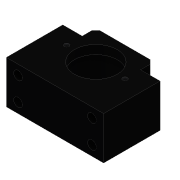
# Autodesk Inventor part: Lagerbock_Loslager
Saved by Autodesk Inventor 2016 (Build 200138000, 138)
## iProperties
Created: 2015-07-24
Part Number: Lagerbock_Loslager
Material: Aluminum 6061
Document SubType Name: Modeling
Density: 2.71 g/cm^3
Appearance: Smooth - Black
Autodesk Inventor part; units mm, degrees
ref_plane "YZ Plane" through (0, 0, 0) normal (1, 0, 0) x (0, 1, 0)
ref_plane "XZ Plane" through (0, 0, 0) normal (0, 1, 0) x (-1, 0, 0)
ref_plane "XY Plane" through (0, 0, 0) normal (0, 0, 1) x (1, 0, 0)
sketch "Sketch1" plane through (0, 0, 0) normal (0, 0, 1) x (1, 0, 0)
  line L0 (-25, 0) -> (25, 0)
  line L1 (25, 0) -> (25, 29)
  line L2 (25, 29) -> (15, 29)
  line L3 (15, 29) -> (15, 36)
  line L4 (15, 36) -> (-15, 36)
  line L5 (-15, 36) -> (-15, 29)
  line L6 (-15, 29) -> (-25, 29)
  line L7 (-25, 29) -> (-25, 0)
  point P0 (0, 0)
  point P1 (0, 0)
  dimension "d0" = 50
  dimension "d1" = 36
  dimension "d2" = 7
  dimension "d3" = 30
  constraints: 16 end point, 6 perpendicular, 2 point on line, 1 coincident, 1 collinear, 1 horizontal, 1 midpoint
  measures "d0" distance between parallel lines of L1 L7
  measures "d1" distance between parallel lines of L0 L4
  measures "d2" distance between parallel lines of L6 L4
  measures "d3" distance of L3.end L4.end
extrude "Extrusion1" add sketch "Sketch1" along normal mid plane 22
sketch "Sketch2" plane through (0, 0, 11) normal (0, 0, 1) x (1, 0, 0)
  line L0 (-25, 0) -> (25, 0) projected
  point P0 (0, 0)
  point P1 (0, 21)
  point P2 (0, 0)
  dimension "d6" = 21
  constraints: 1 midpoint, 1 vertical alignment
  measures "d6" distance from line of L0 point (0, 21)
hole "Hole1" at (0, 21, 11) direction (0, 0, -1) diameter 22 end through all
chamfer "Chamfer2" distance 2 angle 45 2 edges at (-15, 36, 0) (15, 36, 0)
sketch "Sketch3" plane through (-25, 29, 11) normal (0, 1, 0) x (1, 0, 0)
  line L0 (0, 22) -> (0, 0) projected
  line L1 (50, 22) -> (50, 0) projected
  line L2 (50, 22) -> (0, 22) projected
  line L3 (0, 0) -> (50, 0) projected
  point P0 (25, 11)
  point P1 (6, 17)
  point P2 (44, 17)
  point P3 (6, 5)
  point P4 (44, 5)
  dimension "d20" = 38
  dimension "d21" = 6
  dimension "d22" = 6
  dimension "d49" = 12
  dimension "d50" = 5
  dimension "d51" = 5
  constraints: 2 horizontal alignment, 2 vertical alignment
  measures "d20" distance of point (44, 17) point (6, 17)
  measures "d21" distance from line of L0 point (6, 17)
  measures "d22" distance from line of L1 point (44, 17)
  measures "d49" distance of point (6, 5) point (6, 17)
  measures "d50" distance from line of L2 point (6, 17)
  measures "d51" distance from line of L3 point (6, 5)
hole "Hole2" at (-19, 29, -6) at (19, 29, -6) at (-19, 29, 6) at (19, 29, 6) direction (0, -1, 0) diameter 4.5 end through all counterbore diameter 8 counterbore depth 5
sketch "Sketch5" plane through (0, 0, 11) normal (0, 0, 1) x (1, 0, 0)
  circle A0 centre (0, 21) radius 11 projected
  point P0 (0, 0)
  point P1 (-15, 21)
  point P2 (15, 21)
  dimension "d40" = 30
  dimension "d52" = 15
  constraints: 1 centre point, 1 horizontal alignment
  measures "d40" distance of point (15, 21) point (-15, 21)
  measures "d52" distance of point (15, 21) A0.centre
hole "Hole4" at (-15, 21, 11) at (15, 21, 11) direction (0, 0, -1) diameter 2.459 depth 10 tip angle 118 thread size "M3x0.5" designation "M3" class "6H" standard "ISO Metric profile"
hole "Hole5" at (0, 21, -11) direction (0, 0, 1) diameter 26 depth 17.5
sketch "Sketch6" plane through (0, 0, -11) normal (0, 0, -1) x (-1, 0, 0)
  circle A0 centre (0, 21) radius 15.5563 construction
  circle A1 centre (0, 21) radius 13 construction
  point P0 (0, 0)
  point P1 (-11, 32)
  point P2 (-11, 10)
  point P3 (11, 10)
  point P4 (11, 32)
  dimension "d62" = 22
  dimension "d63" = 22
  constraints: 4 point on circle, 2 horizontal alignment, 2 vertical alignment, 1 centre point, 1 concentric
  measures "d62" distance of A0.end A0.start
  measures "d63" distance of point (11, 32) A0.start
hole "Hole6" at (11, 32, -11) at (11, 10, -11) at (-11, 10, -11) at (-11, 32, -11) direction (0, 0, 1) diameter 2.459 depth 8 tip angle 118 thread size "M3x0.5" class "6H" standard "ISO Metric profile"
equation "\"d52\" = 0.5 * d40"
body "Solid1"
